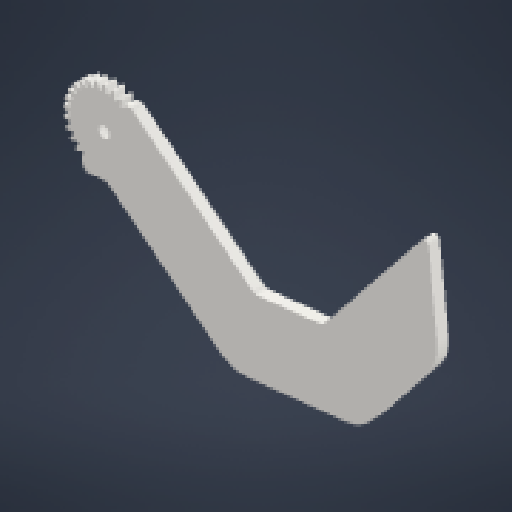
# Autodesk Inventor part: Engranaje recto2
Saved by Autodesk Inventor 2026.3 (Build 303398000, 398)
## iProperties
CustomPartVersion: 1
Created: 2026-04-16
Part Number: Engranaje recto2
Material: Steel
Document SubType Name: Modeling
Designer: Jose Carlos
Categories: <?xml version="1.0" encoding="UTF-16"?> <MemberInstance><Categories><FamilyTemplate><FamilyTemplateParameter ValueType="xs:double" Id="1" ObjectReferenceKey="da_z" ObjectType="kUserParameterObject"/><FamilyTemplateParameter ValueType="xs:double" Id="2" ObjectReferenceKey="da_b" ObjectType="kUserParameterObject"/><FamilyTemplateParameter ValueType="xs:double" Id="3" ObjectReferenceKey="da_beta" ObjectType="kUserParameterObject"/><FamilyTemplateParameter ValueType="xs:double" Id="4" ObjectReferenceKey="da_da" ObjectType="kUserParameterObject"/><FamilyTemplateParameter ValueType="xs:double" Id="5" ObjectReferenceKey="da_aw" ObjectType="kUserParameterObject"/><FamilyTemplateParameter ValueType="xs:string" Id="6" ObjectReferenceKey="EAIAABAAAACIAQAAAAAAAIAAAAAAAAAA" ObjectType="83910656" SubObjectId="SurfaceGeometry"/></FamilyTemplate><ParamToTemplateMap><ParamToTemplate CategoryParameter="//CategoryParameter[@InternalName='046C89C9-8512-4d59-83FE-43B91F4F132A']" TemplateParameter="1"/><ParamToTemplate CategoryParameter="//CategoryParameter[@InternalName='2552DF32-E462-4b46-AEBF-C6C7768E72AC']" TemplateParameter="2"/><ParamToTemplate CategoryParameter="//CategoryParameter[@InternalName='C9EE641D-15FC-4fae-A226-E94C4372FDD7']" TemplateParameter="3"/><ParamToTemplate><ParamToTemplate CategoryParameter="//CategoryParameter[@InternalName='00B6519A-459B-49c7-AD84-2E56D39A5744']" ConstantValue="0.072098"/></ParamToTemplate><ParamToTemplate><ParamToTemplate CategoryParameter="//CategoryParameter[@InternalName='04B31F0E-C7A6-4894-AA32-9629BEFACF47']" ConstantValue="1.000000"/></ParamToTemplate><ParamToTemplate><ParamToTemplate CategoryParameter="//CategoryParameter[@InternalName='43CBEC2E-7847-49e7-A936-2F7889FCB2D9']" ConstantValue="0.250000"/></ParamToTemplate><ParamToTemplate><ParamToTemplate CategoryParameter="//CategoryParameter[@InternalName='B1EFC894-105D-4ebd-86BF-FA20ED196853']" ConstantValue="0.350000"/></ParamToTemplate><ParamToTemplate><ParamToTemplate CategoryParameter="//CategoryParameter[@InternalName='51175063-3D10-4879-93E8-6246FE8B403D']" ConstantValue="2060000000.000000"/></ParamToTemplate><ParamToTemplate><ParamToTemplate CategoryParameter="//CategoryParameter[@InternalName='A3A52E27-4454-46a9-B0BD-C932399B70AF']" ConstantValue="0.300000"/></ParamToTemplate><ParamToTemplate><ParamToTemplate CategoryParameter="//CategoryParameter[@InternalName='91B76062-C214-41d9-B1B9-14D2AB99603D']" ConstantValue="0.070000"/></ParamToTemplate><ParamToTemplate><ParamToTemplate CategoryParameter="//CategoryParameter[@InternalName='374E806E-8B8A-4dda-A9AA-1039D6500AD2']" ConstantValue="14.285714"/></ParamToTemplate><ParamToTemplate><ParamToTemplate CategoryParameter="//CategoryParameter[@InternalName='2D373A89-B862-43d6-8D0B-0CBF12AB9F6C']" ConstantValue="0.349066"/></ParamToTemplate><ParamToTemplate CategoryParameter="//CategoryParameter[@InternalName='37777632-D6A2-4fac-9D53-DB8ACD95C989']" TemplateParameter="4"/><ParamToTemplate CategoryParameter="//CategoryParameter[@InternalName='FD1017F1-B727-4f7e-9707-0F86F1FF9423']" TemplateParameter="5"/><ParamToTemplate><ParamToTemplate CategoryParameter="//CategoryParameter[@InternalName='9E1B4470-B2D3-4ff1-B813-535BB4CDF51A']" ConstantValue="3520000.000000"/></ParamToTemplate><ParamToTemplate><ParamToTemplate CategoryParameter="//CategoryParameter[@InternalName='F8452263-BFF6-458c-9FB1-07C4B99E95CD']" ConstantValue="11400000.000000"/></ParamToTemplate><ParamToTemplate><ParamToTemplate CategoryParameter="//CategoryParameter[@InternalName='3E3BB259-FD49-497f-8171-6EBC954A3479']" ConstantValue="2.000000"/></ParamToTemplate><ParamToTemplate CategoryParameter="//CategoryParameter[@InternalName='27C3BAF2-7550-4e4b-AE2C-0DB134B7D9B7']" TemplateParameter="6"/></ParamToTemplateMap><Category DisplayName="Gear" InternalName="DC85795E-93AB-48d5-8EEE-5A27447B64BD" Mnemonic="Gear"><CategoryParameter DisplayName="z" InternalName="046C89C9-8512-4d59-83FE-43B91F4F132A" Mnemonic="z"/><CategoryParameter DisplayName="b" InternalName="2552DF32-E462-4b46-AEBF-C6C7768E72AC" Mnemonic="b"/><CategoryParameter DisplayName="||b|" InternalName="C9EE641D-15FC-4fae-A226-E94C4372FDD7" Mnemonic="beta"/><CategoryParameter DisplayName="x" InternalName="00B6519A-459B-49c7-AD84-2E56D39A5744" Mnemonic="x"/><CategoryParameter DisplayName="a*" InternalName="04B31F0E-C7A6-4894-AA32-9629BEFACF47" Mnemonic="a"/><CategoryParameter DisplayName="c*" InternalName="43CBEC2E-7847-49e7-A936-2F7889FCB2D9" Mnemonic="c"/><CategoryParameter DisplayName="r|.f|*" InternalName="B1EFC894-105D-4ebd-86BF-FA20ED196853" Mnemonic="rf"/><CategoryParameter DisplayName="E" InternalName="51175063-3D10-4879-93E8-6246FE8B403D" Mnemonic="E"/><CategoryParameter DisplayName="||m|" InternalName="A3A52E27-4454-46a9-B0BD-C932399B70AF" Mnemonic="mi"/><Category DisplayName="SpurGear" InternalName="26C5A22E-A91E-4dfd-A3B3-23CCAFAE1764" Mnemonic="SpurGear"><CategoryParameter DisplayName="m" InternalName="91B76062-C214-41d9-B1B9-14D2AB99603D" Mnemonic="m"/><CategoryParameter DisplayName="P" InternalName="374E806E-8B8A-4dda-A9AA-1039D6500AD2" Mnemonic="PP"/><CategoryParameter DisplayName="||a|" InternalName="2D373A89-B862-43d6-8D0B-0CBF12AB9F6C" Mnemonic="alpha"/><CategoryParameter DisplayName="d|.a|" InternalName="37777632-D6A2-4fac-9D53-DB8ACD95C989" Mnemonic="da"/><CategoryParameter DisplayName="a|.w|" InternalName="FD1017F1-B727-4f7e-9707-0F86F1FF9423" Mnemonic="aw"/><CategoryParameter DisplayName="||s||.Flim|" InternalName="9E1B4470-B2D3-4ff1-B813-535BB4CDF51A" Mnemonic="sFlim"/><CategoryParameter DisplayName="||s||.Hlim|" InternalName="F8452263-BFF6-458c-9FB1-07C4B99E95CD" Mnemonic="sHlim"/><CategoryParameter DisplayName="tipo" InternalName="3E3BB259-FD49-497f-8171-6EBC954A3479" Mnemonic="type"/><CategoryParameter DisplayName="PitchDiameter" InternalName="27C3BAF2-7550-4e4b-AE2C-0DB134B7D9B7" Mnemonic="IDS_PITCHDIAM"/></Category></Category></Categories></MemberInstance>
Density: 1 g/cm^3
Appearance: Steel
Author: Jose Carlos
Autodesk Inventor part; units mm, degrees
sketch "Sketch1" plane through (0, 0, 0) normal (0, 0, 1) x (1, 0, 0)
  circle A0 centre (0, 0) radius 10.9
  dimension "d0" = 21.8
  constraints: 1 centre point
  measures "d0" diameter of A0
extrude "Extrusion1" add sketch "Sketch1" along normal blind 3
ref_plane "Work Plane2" through (0, 0, 1.5) normal (0, 0, 1) x (1, 0, 0)
sketch "Sketch2" plane through (0, 0, 0) normal (0, 0, -1) x (-1, 0, 0)
  circle A0 centre (0, 0) radius 10.9 projected
  circle A1 centre (0, 0) radius 10.15
  dimension "d3" = 20.3
  constraints: 1 centre point, 1 coincident
  measures "d3" diameter of A1
surface extrude "Diámetro de separación" sketch "Sketch2" against normal through all shown no curves A1
ref_plane "Work Plane8" through (0, 0, 0) normal (0.994138, 0.108119, 0) x (0, 0, 1)
ref_plane "Work Plane9" through (0, 0, 0) normal (1, 0, 0) x (0, 1, 0)
spur gear teeth "Engranaje recto" teeth 29 pitch diameter 20.3 tip diameter 21.8 root diameter 18.6509 face width 3 start plane through (0, 0, 0) normal (0, 0, -1) x (-1, 0, 0)
sketch "Boceto3" plane through (0, 0, 0) normal (0, 0, -1) x (-1, 0, 0)
  arc A0 (-20.6399, 61.4908) -> (-27.3528, 65.1671) centre (-28.434, 55.2257) ccw projected
  line L0 (-27.3528, 65.1671) -> (-53.9119, 68.0556) projected
  arc A1 (-53.9119, 68.0556) -> (-61.2582, 65.9083) centre (-54.9931, 58.1142) ccw projected
  line L1 (-61.2582, 65.9083) -> (-80.7523, 50.2386) projected
  arc A2 (-80.7523, 50.2386) -> (-84.4286, 43.5256) centre (-74.4872, 42.4444) ccw projected
  line L2 (-84.4286, 43.5256) -> (-86.7778, 21.9251) projected
  arc A3 (-86.7778, 21.9251) -> (-85.1571, 21.0375) centre (-85.7837, 21.8169) ccw projected
  line L3 (-85.1571, 21.0375) -> (-52.6022, 47.206) projected
  arc A4 (-51.1329, 47.6354) -> (-52.6022, 47.206) centre (-51.3491, 45.6471) ccw projected
  line L4 (-51.1329, 47.6354) -> (-34.4566, 45.8218) projected
  arc A5 (-33.114, 45.0865) -> (-34.4566, 45.8218) centre (-34.6729, 43.8335) ccw projected
  line L5 (-33.114, 45.0865) -> (-7.3906, 13.0851) projected
  arc A6 (-7.3906, 13.0851) -> (-5.2331, 12.4298) centre (-5.8318, 14.3381) ccw projected
  arc A7 (-5.2331, 12.4298) -> (-5.0212, 12.2253) centre (2.1624, 19.8828) ccw projected
  arc A8 (-5.0212, 12.2253) -> (-3.5694, 13.0415) centre (-7.6024, 18.5161) ccw projected
  arc A9 (-3.5694, 13.0415) -> (-3.1767, 12.7309) centre (2.1624, 19.8828) ccw projected
  arc A10 (-3.1767, 12.7309) -> (-3.637, 11.1302) centre (3.0789, 10.0655) ccw projected
  arc A11 (-3.637, 11.1302) -> (-3.1371, 10.8188) centre (2.1624, 19.8828) ccw projected
  arc A12 (-3.1371, 10.8188) -> (-1.9033, 11.9376) centre (-7.0535, 16.3775) ccw projected
  arc A13 (-1.9033, 11.9376) -> (-1.4514, 11.7221) centre (2.1624, 19.8828) ccw projected
  arc A14 (-1.4514, 11.7221) -> (-1.544, 10.0592) centre (5.2405, 10.5156) ccw projected
  arc A15 (-1.544, 10.0592) -> (-0.9874, 9.8668) centre (2.1624, 19.8828) ccw projected
  arc A16 (-0.9874, 9.8668) -> (-0.0334, 11.2321) centre (-6.0424, 14.4147) ccw projected
  arc A17 (-0.0334, 11.2321) -> (0.4551, 11.1226) centre (2.1624, 19.8828) ccw projected
  arc A18 (0.4551, 11.1226) -> (0.7349, 9.4807) centre (7.2477, 11.4354) ccw projected
  arc A19 (0.7349, 9.4807) -> (1.3204, 9.417) centre (2.1624, 19.8828) ccw projected
  arc A20 (1.3204, 9.417) -> (1.9466, 10.9604) centre (-4.62, 12.7261) ccw projected
  arc A21 (1.9466, 10.9604) -> (2.4472, 10.9623) centre (2.1624, 19.8828) ccw projected
  arc A22 (2.4472, 10.9623) -> (3.0853, 9.4239) centre (8.9999, 12.7788) ccw projected
  arc A23 (3.0853, 9.4239) -> (3.6703, 9.4921) centre (2.1624, 19.8828) ccw projected
  arc A24 (3.6703, 9.4921) -> (3.9374, 11.1361) centre (-2.8574, 11.3963) ccw projected
  arc A25 (3.9374, 11.1361) -> (4.4251, 11.2493) centre (2.1624, 19.8828) ccw projected
  arc A26 (4.4251, 11.2493) -> (5.3895, 9.8915) centre (10.4092, 14.4784) ccw projected
  arc A27 (5.3895, 9.8915) -> (5.9447, 10.0881) centre (2.1624, 19.8828) ccw projected
  arc A28 (5.9447, 10.0881) -> (5.8392, 11.7503) centre (-0.8431, 10.4921) ccw projected
  arc A29 (5.8392, 11.7503) -> (6.2894, 11.9693) centre (2.1624, 19.8828) ccw projected
  arc A30 (6.2894, 11.9693) -> (7.5319, 10.8601) centre (11.4051, 16.449) ccw projected
  arc A31 (7.5319, 10.8601) -> (8.0293, 11.1754) centre (2.1624, 19.8828) ccw projected
  arc A32 (8.0293, 11.1754) -> (7.5567, 12.7724) centre (1.3219, 10.0587) ccw projected
  arc A33 (7.5567, 12.7724) -> (7.9469, 13.0861) centre (2.1624, 19.8828) ccw projected
  arc A34 (7.9469, 13.0861) -> (9.405, 12.2811) centre (11.9374, 18.5917) ccw projected
  arc A35 (9.405, 12.2811) -> (9.8198, 12.6992) centre (2.1624, 19.8828) ccw projected
  arc A36 (9.8198, 12.6992) -> (9.0036, 14.151) centre (3.529, 10.118) ccw projected
  arc A37 (9.0036, 14.151) -> (9.3143, 14.5436) centre (2.1624, 19.8828) ccw projected
  arc A38 (9.3143, 14.5436) -> (10.9149, 14.0834) centre (11.9796, 20.7993) ccw projected
  arc A39 (10.9149, 14.0834) -> (11.2263, 14.5832) centre (2.1624, 19.8828) ccw projected
  arc A40 (11.2263, 14.5832) -> (10.1075, 15.8171) centre (5.6676, 10.6669) ccw projected
  arc A41 (10.1075, 15.8171) -> (10.323, 16.2689) centre (2.1624, 19.8828) ccw projected
  arc A42 (10.323, 16.2689) -> (11.986, 16.1764) centre (11.5295, 22.9608) ccw projected
  arc A43 (11.986, 16.1764) -> (12.1783, 16.733) centre (2.1624, 19.8828) ccw projected
  arc A44 (12.1783, 16.733) -> (10.813, 17.687) centre (7.6304, 11.678) ccw projected
  arc A45 (10.813, 17.687) -> (10.9226, 18.1755) centre (2.1624, 19.8828) ccw projected
  arc A46 (10.9226, 18.1755) -> (12.5644, 18.4553) centre (10.6098, 24.968) ccw projected
  arc A47 (12.5644, 18.4553) -> (12.6281, 19.0408) centre (2.1624, 19.8828) ccw projected
  arc A48 (12.6281, 19.0408) -> (11.0848, 19.667) centre (9.3191, 13.1004) ccw projected
  arc A49 (11.0848, 19.667) -> (11.0828, 20.1676) centre (2.1624, 19.8828) ccw projected
  arc A50 (11.0828, 20.1676) -> (12.6213, 20.8057) centre (9.2664, 26.7203) ccw projected
  arc A51 (12.6213, 20.8057) -> (12.5531, 21.3907) centre (2.1624, 19.8828) ccw projected
  arc A52 (12.5531, 21.3907) -> (10.9091, 21.6578) centre (10.6488, 14.863) ccw projected
  arc A53 (10.9091, 21.6578) -> (10.7958, 22.1454) centre (2.1624, 19.8828) ccw projected
  arc A54 (10.7958, 22.1454) -> (12.1537, 23.1099) centre (7.5668, 28.1296) ccw projected
  arc A55 (12.1537, 23.1099) -> (11.957, 23.665) centre (2.1624, 19.8828) ccw projected
  arc A56 (11.957, 23.665) -> (10.2948, 23.5596) centre (11.5531, 16.8773) ccw projected
  arc A57 (10.2948, 23.5596) -> (10.0758, 24.0098) centre (2.1624, 19.8828) ccw projected
  arc A58 (10.0758, 24.0098) -> (11.1851, 25.2523) centre (5.5962, 29.1254) ccw projected
  arc A59 (11.1851, 25.2523) -> (10.8698, 25.7497) centre (2.1624, 19.8828) ccw projected
  arc A60 (10.8698, 25.7497) -> (9.2727, 25.2771) centre (11.9864, 19.0422) ccw projected
  arc A61 (9.2727, 25.2771) -> (8.9591, 25.6673) centre (2.1624, 19.8828) ccw projected
  arc A62 (8.9591, 25.6673) -> (9.764, 27.1254) centre (3.4534, 29.6578) ccw projected
  arc A63 (9.764, 27.1254) -> (9.5579, 27.3357) centre (2.1624, 19.8828) ccw projected
  arc A64 (9.5579, 27.3357) -> (8.1603, 30.5054) centre (7.9441, 28.5171) ccw projected
  line L6 (8.1603, 30.5054) -> (4.7175, 30.8798) projected
  arc A65 (3.3749, 31.6151) -> (4.7175, 30.8798) centre (4.9337, 32.8681) ccw projected
  line L7 (3.3749, 31.6151) -> (-20.6399, 61.4908) projected
  arc A66 (3.4461, 18.7373) -> (3.0052, 18.3828) centre (3.4028, 18.3396) ccw projected
  line L8 (3.0052, 18.3828) -> (2.8862, 17.2893) projected
  line L9 (2.8862, 17.2893) -> (0.8979, 17.5055) projected
  line L10 (0.8979, 17.5055) -> (1.0169, 18.5991) projected
  arc A67 (1.0169, 18.5991) -> (0.6625, 19.04) centre (0.6192, 18.6423) ccw projected
  line L11 (0.6625, 19.04) -> (-0.4311, 19.1589) projected
  line L12 (-0.4311, 19.1589) -> (-0.2148, 21.1472) projected
  line L13 (-0.2148, 21.1472) -> (0.8787, 21.0283) projected
  arc A68 (0.8787, 21.0283) -> (1.3196, 21.3827) centre (0.922, 21.4259) ccw projected
  line L14 (1.3196, 21.3827) -> (1.4385, 22.4762) projected
  line L15 (1.4385, 22.4762) -> (3.4268, 22.26) projected
  line L16 (3.4268, 22.26) -> (3.3079, 21.1664) projected
  arc A69 (3.3079, 21.1664) -> (3.6623, 20.7255) centre (3.7055, 21.1232) ccw projected
  line L17 (3.6623, 20.7255) -> (4.7558, 20.6066) projected
  line L18 (4.7558, 20.6066) -> (4.5396, 18.6183) projected
  line L19 (4.5396, 18.6183) -> (3.4461, 18.7373) projected
  line L20 (9.5579, 27.3357) -> (-5.2331, 12.4298)
  line L21 (-23.7723, 12.6444) -> (-80.0092, 18.7605) construction
  arc A70 (-38.56, -37.8807) -> (-31.2137, -35.7335) centre (-37.4788, -27.9393) ccw
  line L22 (-38.56, -37.8807) -> (-65.1191, -34.9922)
  arc A71 (-71.832, -31.316) -> (-65.1191, -34.9922) centre (-64.0379, -25.0509) ccw
  line L23 (-71.832, -31.316) -> (-87.5018, -11.8219)
  arc A72 (-89.649, -4.4756) -> (-87.5018, -11.8219) centre (-79.7077, -5.5568) ccw
  line L24 (-89.649, -4.4756) -> (-87.2998, 17.1249)
  arc A73 (-85.5263, 17.6433) -> (-87.2998, 17.1249) centre (-86.3057, 17.0168) ccw
  line L25 (-85.5263, 17.6433) -> (-59.3579, -14.9116)
  arc A74 (-59.3579, -14.9116) -> (-58.0153, -15.6469) centre (-57.799, -13.6586) ccw
  line L26 (-58.0153, -15.6469) -> (-41.339, -17.4606)
  arc A75 (-41.339, -17.4606) -> (-39.8697, -17.0311) centre (-41.1228, -15.4723) ccw
  line L27 (-39.8697, -17.0311) -> (-7.8683, 8.6923)
  arc A76 (-5.6204, 8.8685) -> (-7.8683, 8.6923) centre (-6.6153, 7.1335) ccw
  arc A77 (-5.3695, 9.0227) -> (-5.6204, 8.8685) centre (0, 0) ccw
  arc A78 (-4.1271, 7.9135) -> (-5.3695, 9.0227) centre (-9.2427, 3.4338) ccw
  arc A79 (-3.6769, 8.1324) -> (-4.1271, 7.9135) centre (0, 0) ccw
  arc A80 (-1.775, 8.7467) -> (-2.2627, 8.6334) centre (0, 0) ccw
  arc A81 (3.5742, -11.6637) -> (5.6204, -8.8685) centre (3.7904, -9.6754) ccw
  line L28 (3.5742, -11.6637) -> (0.1313, -11.2892)
  arc A82 (0.1313, -11.2892) -> (-1.3379, -11.7187) centre (-0.0849, -13.2775) ccw
  line L29 (-1.3379, -11.7187) -> (-31.2137, -35.7335)
  line L30 (5.6204, -8.8685) -> (-5.6204, 8.8685)
  point P0 (-8.2469, 5.4044)
  point P1 (-6.8375, 7.104)
  point P2 (6.7823, 7.1567)
  point P3 (-5.0853, 8.4474)
  point P4 (8.2048, 5.468)
  point P5 (-3.0781, 9.3672)
  point P6 (9.2158, 3.5052)
  point P7 (5.7994, 8.7525)
  point P8 (5.3391, 7.1519)
  point P9 (5.7317, 6.8413)
  point P10 (7.1836, 7.6574)
  point P11 (9.7648, 1.3666)
  point P12 (7.6016, 7.2426)
  point P13 (6.7967, 5.7845)
  point P14 (7.1104, 5.3943)
  point P15 (8.7074, 5.867)
  point P16 (9.824, -0.8405)
  point P17 (9.0227, 5.3695)
  point P18 (7.9135, 4.1271)
  point P19 (8.1324, 3.6769)
  point P20 (9.7946, 3.7823)
  point P21 (9.3907, -3.0055)
  point P22 (9.9913, 3.2271)
  point P23 (8.6334, 2.2627)
  point P24 (8.7467, 1.775)
  point P25 (10.3907, 1.5079)
  point P26 (8.4865, -5.0198)
  point P27 (10.4589, 0.923)
  point P28 (7.104, 6.8375)
  point P29 (8.9224, -0.2158)
  point P30 (10.4657, -0.842)
  point P31 (10.402, -1.4275)
  point P32 (8.7602, -1.7073)
  point P33 (8.4474, 5.0853)
  point P34 (8.6507, -2.1958)
  point P35 (10.016, -3.1497)
  point P36 (5.468, -8.2048)
  point P37 (9.8236, -3.7064)
  point P38 (8.1606, -3.6138)
  point P39 (9.3672, 3.0781)
  point P40 (7.9452, -4.0657)
  point P41 (9.064, -5.2995)
  point P42 (3.5052, -9.2158)
  point P43 (8.7525, -5.7994)
  point P44 (7.1519, -5.3391)
  point P45 (9.8172, 0.9165)
  point P46 (6.8413, -5.7317)
  point P47 (7.6574, -7.1836)
  point P48 (1.3666, -9.7648)
  point P49 (5.7845, -6.7967)
  point P50 (9.775, -1.291)
  point P51 (5.3943, -7.1104)
  point P52 (5.867, -8.7074)
  point P53 (-0.8405, -9.824)
  point P54 (1.1455, 1.2837)
  point P55 (1.4999, 0.8428)
  point P56 (1.5432, 1.2404)
  point P57 (1.2644, 2.3772)
  point P58 (-0.7238, 2.5935)
  point P59 (-0.8428, 1.4999)
  point P60 (-1.2837, 1.1455)
  point P61 (-1.2404, 1.5432)
  point P62 (-2.3772, 1.2644)
  point P63 (-2.5935, -0.7238)
  point P64 (-1.4999, -0.8428)
  point P65 (-1.1455, -1.2837)
  point P66 (-1.5432, -1.2404)
  point P67 (-1.2644, -2.3772)
  point P68 (0.7238, -2.5935)
  point P69 (0.8428, -1.4999)
  point P70 (1.2837, -1.1455)
  point P71 (1.2404, -1.5432)
  point P72 (2.3772, -1.2644)
  point P73 (2.5935, 0.7238)
  constraints: 136 symmetric about line, 26 point on circle, 20 end point, 13 centre point, 13 other
extrude "Extrusión2" add sketch "Boceto3" against normal up to surface (3 mm away) contours L22 A71 L23 A72 L24 A73 L25 A74 L26 A75 L27 A76 L30 A81 L28 A82 L29 A70
sketch "Boceto4" plane through (0, 0, 0) normal (0, 0, -1) x (-1, 0, 0)
  point P0 (0, 0)
  point P1 (0, 0)
  constraints: 1 coincident
hole "Agujero1" at (0, 0, 0) direction (0, 0, 1) diameter 3 end through all
equation "\"d0\" = da_da"
equation "\"d1\" = da_b"
equation "\"d3\" = da_d"
equation "\"da_da\" = 21.8"
equation "\"da_b\" = 3"
equation "\"da_d\" = 20.3"
body "Solid1"
body "Srf1"
